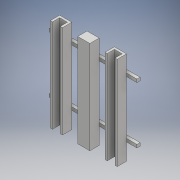
# Autodesk Inventor part: tracks
Saved by Autodesk Inventor 2018 (Build 220112000, 112)
## iProperties
Created: 2017-12-09
Part Number: tracks
Material: Generic
Document SubType Name: Modeling
Designer: ragna
Density: 1 g/cm^3
Appearance: Default
Author: ragna
Autodesk Inventor part; units mm, degrees
ref_plane "YZ Plane" through (0, 0, 0) normal (1, 0, 0) x (0, 1, 0)
ref_plane "XZ Plane" through (0, 0, 0) normal (0, 1, 0) x (-1, 0, 0)
sketch "Sketch1" plane through (0, 0, 0) normal (0, 1, 0) x (-1, 0, 0)
  line L0 (0, 0) -> (-11.7, 0)
  line L1 (-11.7, 0) -> (-11.7, -89.46)
  line L2 (-11.7, -89.46) -> (0, -89.46)
  line L3 (0, -89.46) -> (0, 0)
  line L4 (-26.35, 0) -> (-38.05, 0)
  line L5 (-38.05, 0) -> (-38.05, -89.46)
  line L6 (-38.05, -89.46) -> (-26.35, -89.46)
  line L7 (-26.35, -89.46) -> (-26.35, 0)
  line L8 (-52.7, 0) -> (-64.4, 0)
  line L9 (-64.4, 0) -> (-64.4, -89.46)
  line L10 (-64.4, -89.46) -> (-52.7, -89.46)
  line L11 (-52.7, -89.46) -> (-52.7, 0)
  dimension "d0" = 11.7
  dimension "d1" = 11.7
  dimension "d2" = 11.7
  dimension "d3" = 14.65
  dimension "d4" = 14.65
  dimension "d5" = 89.46
  dimension "d47" = 64.4
  constraints: 24 end point, 6 parallel, 4 point on line, 3 horizontal, 3 perpendicular, 1 coincident
  measures "d0" distance of L1.end L2.end
  measures "d1" distance of L5.end L6.end
  measures "d2" distance of L9.end L10.end
  measures "d3" distance between parallel lines of L7 L1
  measures "d4" distance between parallel lines of L11 L5
  measures "d5" distance of L2.end L0.start
  measures "d47" distance between parallel lines of L9 L3
extrude "Extrusion1" add sketch "Sketch1" along normal blind 9
sketch "Sketch2" plane through (0, 9, 0) normal (0, 1, 0) x (1, 0, 0)
  line L0 (38.05, 89.46) -> (26.35, 89.46) construction
  line L1 (32.2, 89.46) -> (32.2, 0) construction
  line L2 (26.35, 0) -> (38.05, 0) construction
  line L3 (11.7, 89.46) -> (0, 89.46) construction
  line L4 (5.85, 89.46) -> (5.85, 0) construction
  line L5 (0, 0) -> (11.7, 0) construction
  circle A0 centre (5.85, 84.96) radius 1.5
  circle A1 centre (58.55, 84.96) radius 1.5
  dimension "d8" = 3
  dimension "d9" = 4.5
  constraints: 4 end point, 4 midpoint, 2 centre point, 1 point on line, 1 symmetric about line, 1 other
  measures "d8" diameter of A0
  measures "d9" distance from line of L3 A0.centre
extrude "Extrusion2" cut sketch "Sketch2" against normal blind 8
sketch "Sketch3" plane through (11.7, 0, -89.46) normal (0, 0, -1) x (-1, 0, 0)
  line L0 (-14.65, 9) -> (-26.35, 9) construction
  line L1 (-20.5, 9) -> (-20.5, 0) construction
  line L2 (-14.65, 0) -> (-26.35, 0) construction
  line L3 (0, 0) -> (11.7, 0) projected
  line L4 (9.6, 0) -> (9.6, 6.9)
  line L5 (9.6, 6.9) -> (2.1, 6.9)
  line L6 (2.1, 6.9) -> (2.1, 0)
  line L7 (2.1, 0) -> (9.6, 0) construction
  line L8 (0, 0) -> (0, 9) construction
  line L9 (11.7, 0) -> (11.7, 9) construction
  line L10 (-41, 0) -> (-52.7, 0)
  line L11 (-50.6, 0) -> (-50.6, 6.9)
  line L12 (-50.6, 6.9) -> (-43.1, 6.9)
  line L13 (-43.1, 6.9) -> (-43.1, 0)
  dimension "d15" = 7.5
  dimension "d16" = 2.1
  dimension "d17" = 2.1
  dimension "d18" = 6.9
  constraints: 18 end point, 6 symmetric about line, 4 point on line, 3 perpendicular, 2 midpoint, 1 vertical
  measures "d15" distance between parallel lines of L6 L4
  measures "d16" distance between parallel lines of L8 L6
  measures "d17" distance between parallel lines of L4 L9
  measures "d18" distance between parallel lines of L3 L5
extrude "Extrusion3" cut sketch "Sketch3" against normal through all
sketch "Sketch4" plane through (0, 9, 0) normal (0, 1, 0) x (1, 0, 0)
  line L0 (0, 89.46) -> (0, 0) construction
  line L1 (0, 44.73) -> (64.4, 44.73) construction
  line L2 (64.4, 0) -> (64.4, 89.46) construction
  line L3 (-10, 16) -> (74.4, 16)
  line L4 (74.4, 16) -> (74.4, 19)
  line L5 (74.4, 19) -> (-10, 19)
  line L6 (-10, 19) -> (-10, 16)
  line L7 (-10, 73.46) -> (74.4, 73.46)
  line L8 (74.4, 73.46) -> (74.4, 70.46)
  line L9 (74.4, 70.46) -> (-10, 70.46)
  line L10 (-10, 70.46) -> (-10, 73.46)
  line L11 (52.7, 0) -> (64.4, 0) projected
  dimension "d21" = 3
  dimension "d22" = 10
  dimension "d23" = 10
  dimension "d46" = 16
  constraints: 18 end point, 4 symmetric about line, 2 midpoint, 2 parallel, 1 horizontal, 1 perpendicular
  measures "d21" distance of L4.end L3.end
  measures "d22" distance between parallel lines of L0 L6
  measures "d23" distance between parallel lines of L2 L4
  measures "d46" distance between parallel lines of L3 L11
extrude "Extrusion4" add sketch "Sketch4" along normal blind 3
ref_plane "Work Plane2" through (32.2, 0, -89.46) normal (-1, 0, 0) x (0, 0, 1)
sketch "Sketch5" plane through (0, 8.5, 0) normal (0, -1, 0) x (1, 0, 0)
  line L0 (23, -75) -> (14, -75)
  line L1 (14, -75) -> (14, -22)
  line L2 (14, -22) -> (23, -22)
  line L3 (23, -22) -> (23, -75)
  line L4 (26, -90) -> (26, 0) projected
  line L5 (11, 0) -> (11, -90) projected
  line L6 (11, -22) -> (26, -22) projected
  line L7 (11, -68) -> (26, -68) projected
  point P0 (0, 0)
  point P1 (18.5, -22)
  dimension "d27" = 3
  dimension "d28" = 3
  dimension "d29" = 9
  dimension "d30" = 7
  constraints: 8 end point, 2 midpoint, 2 parallel, 1 horizontal, 1 perpendicular
  measures "d27" distance between parallel lines of L4 L3
  measures "d28" distance between parallel lines of L5 L1
  measures "d29" distance between parallel lines of L3 L1
  measures "d30" distance between parallel lines of L7 L0
sketch "Sketch6" plane through (23, 8.5, -75) normal (0, 0, -1) x (-1, 0, 0)
  line L0 (9, 0) -> (9, -2) projected
  line L1 (0, 0) -> (0, -2) projected
  line L2 (9, -0.5) -> (0, -0.5)
  line L3 (0, -0.5) -> (0, -1.5)
  line L4 (0, -1.5) -> (9, -1.5)
  line L5 (9, -1.5) -> (9, -0.5)
  line L6 (9, 0) -> (0, 0) projected
  line L7 (9, -2) -> (0, -2) projected
  point P0 (23, -8.5)
  dimension "d34" = 0.5
  dimension "d35" = 0.5
  dimension "d36" = 1
  constraints: 8 end point, 2 parallel, 2 point on line, 1 horizontal, 1 perpendicular
  measures "d34" distance between parallel lines of L6 L2
  measures "d35" distance between parallel lines of L7 L4
  measures "d36" distance between parallel lines of L4 L2
sketch "Sketch7" plane through (14, 8, -75) normal (0, 1, 0) x (1, 0, 0)
  line L0 (1.5, 2) -> (7.5, 2)
  line L1 (7.5, 2) -> (7.5, 4.5)
  line L2 (7.5, 4.5) -> (1.5, 4.5)
  line L3 (1.5, 4.5) -> (1.5, 2)
  line L4 (0, 0) -> (0, 7) projected
  line L5 (9, 0) -> (9, 7) projected
  line L6 (0, 7) -> (9, 7) projected
  point P0 (-14, -75)
  dimension "d39" = 6
  dimension "d40" = 2.5
  dimension "d41" = 1.5
  dimension "d42" = 1.5
  dimension "d43" = 2.5
  constraints: 8 end point, 2 parallel, 1 horizontal, 1 perpendicular
  measures "d39" distance of L2.end L1.end
  measures "d40" distance of L1.end L0.end
  measures "d41" distance between parallel lines of L4 L3
  measures "d42" distance between parallel lines of L5 L1
  measures "d43" distance between parallel lines of L6 L2
equation "\"d1\" = d0"
equation "\"d2\" = d1"
equation "\"d4\" = d3"
equation "\"d17\" = d16"
equation "\"d23\" = d22"
equation "\"d28\" = d27"
equation "\"d35\" = d34"
equation "\"d42\" = d41"
body "Solid1"
